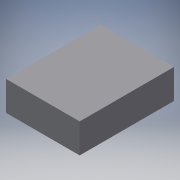
# Autodesk Inventor part: FPGA
Saved by Autodesk Inventor 2019 (Build 230136000, 136)
## iProperties
Created: 2019-03-06
Part Number: FPGA
Material: Generic
Document SubType Name: Modeling
Designer: alarr
Density: 1 g/cm^3
Appearance: Default
Author: alarr
Autodesk Inventor part; units mm, degrees
ref_plane "YZ Plane" through (0, 0, 0) normal (1, 0, 0) x (0, 1, 0)
ref_plane "XZ Plane" through (0, 0, 0) normal (0, 1, 0) x (-1, 0, 0)
ref_plane "XY Plane" through (0, 0, 0) normal (0, 0, 1) x (1, 0, 0)
sketch "Sketch1" plane through (0, 0, 0) normal (0, 1, 0) x (-1, 0, 0)
  line L0 (-31.75, 40.64) -> (31.75, 40.64)
  line L1 (31.75, 40.64) -> (31.75, -40.64)
  line L2 (31.75, -40.64) -> (-31.75, -40.64)
  line L3 (-31.75, -40.64) -> (-31.75, 40.64)
  line L4 (-31.75, 40.64) -> (31.75, -40.64) construction
  line L5 (31.75, 40.64) -> (-31.75, -40.64) construction
  point P0 (0, 0)
  dimension "d0" = 63.5
  dimension "d1" = 81.28
  constraints: 12 end point, 2 midpoint, 2 parallel, 1 horizontal, 1 perpendicular
  measures "d0" distance of L1.end L2.end
  measures "d1" distance of L0.end L1.end
extrude "Extrusion1" add sketch "Sketch1" along normal blind 25.4
body "Solid1"
